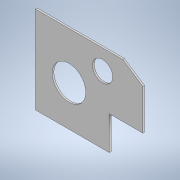
# Autodesk Inventor part: Assignment 4.2 - Spacer Plate
Saved by Autodesk Inventor 2022 (Build 260153000, 153)
## iProperties
Created: 2021-05-24
Part Number: Assignment 4.2 - Spacer Plate
Material: Generic
Document SubType Name: Modeling
Designer: Aaron
Density: 1 g/cm^3
Appearance: Default
Author: Aaron
Autodesk Inventor part; units mm, degrees
ref_plane "YZ Plane" through (0, 0, 0) normal (1, 0, 0) x (0, 1, 0)
ref_plane "XZ Plane" through (0, 0, 0) normal (0, 1, 0) x (-1, 0, 0)
ref_plane "XY Plane" through (0, 0, 0) normal (0, 0, 1) x (1, 0, 0)
sketch "Sketch1" plane through (0, 0, 0) normal (0, 0, 1) x (1, 0, 0)
  line L0 (0, 0) -> (139.7, 0)
  line L1 (139.7, 0) -> (139.7, 63.5)
  line L2 (139.7, 63.5) -> (203.2, 63.5)
  line L3 (203.2, 63.5) -> (203.2, 139.7)
  line L4 (0, 0) -> (0, 165.1)
  line L5 (0, 165.1) -> (165.1, 165.1)
  line L6 (165.1, 165.1) -> (203.2, 139.7)
  circle A0 centre (63.5, 76.2) radius 31.75
  circle A1 centre (127, 127) radius 19.05
  dimension "d0" = 139.7
  dimension "d1" = 63.5
  dimension "d2" = 63.5
  dimension "d3" = 76.2
  dimension "d4" = 165.1
  dimension "d5" = 165.1
  dimension "d8" = 63.5
  dimension "d11" = 38.1
  constraints: 14 end point, 4 perpendicular, 2 centre point, 1 horizontal, 1 vertical
  measures "d0" distance of L0.start L0.end
  measures "d1" distance of L0.end L1.end
  measures "d2" distance of L1.end L2.end
  measures "d3" distance of L2.end L3.end
  measures "d4" distance of L0.start L4.end
  measures "d5" distance of L4.end L5.end
  measures "d8" diameter of A0
  measures "d11" diameter of A1
extrude "Extrusion1" add sketch "Sketch1" against normal blind 3.175
body "Solid1"
